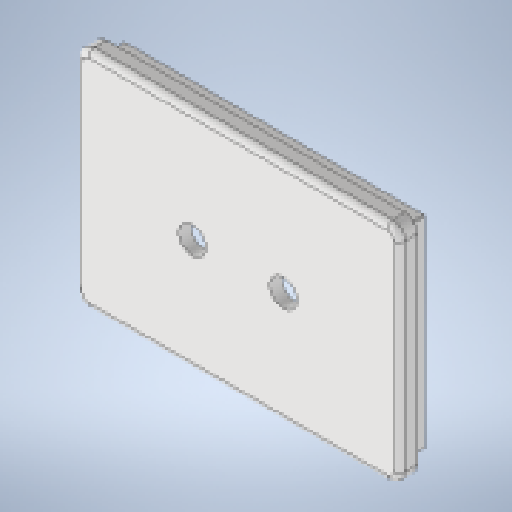
# Autodesk Inventor part: Frame_Bottom
Saved by Autodesk Inventor 2023 (Build 270158000, 158)
## iProperties
Created: 2023-10-08
Part Number: Frame_Bottom
Material: Generic
Document SubType Name: Modeling
Designer: a laptop
Density: 1 g/cm^3
Appearance: Default
Author: a laptop
Autodesk Inventor part; units mm, degrees
ref_plane "YZ Plane" through (0, 0, 0) normal (1, 0, 0) x (0, 1, 0)
ref_plane "XZ Plane" through (0, 0, 0) normal (0, 1, 0) x (-1, 0, 0)
ref_plane "XY Plane" through (0, 0, 0) normal (0, 0, 1) x (1, 0, 0)
sketch "Sketch1" plane through (0, 0, 0) normal (0, 0, 1) x (1, 0, 0)
  circle A0 centre (5, 5) radius 2.35
  line L0 (0, 0) -> (53.18, 0)
  line L1 (53.18, 0) -> (53.18, 36.924)
  line L2 (53.18, 36.924) -> (0, 36.924)
  line L3 (0, 36.924) -> (0, 0)
  circle A1 centre (5, 31.924) radius 2.35
  circle A2 centre (48.18, 5) radius 2.35
  circle A3 centre (48.18, 31.924) radius 2.35
  dimension "d0" = 5
  dimension "d1" = 5
  dimension "d4" = 26.924
  dimension "d7" = 43.18
  dimension "d10" = 5
  dimension "d11" = 5
  dimension "d12" = 4.7
  constraints: 8 end point, 4 centre point, 2 horizontal, 2 parallel, 1 perpendicular, 1 vertical, 6 other
  measures "d0" horizontal distance of L0.start A0.centre
  measures "d1" horizontal distance of L0.start A0.centre
  measures "d4" distance of A0.centre A1.centre
  measures "d7" distance of A0.centre A2.centre
  measures "d10" distance from line of L2 A3.centre
  measures "d11" distance from line of A3.centre L1
  measures "d12" diameter of A0
extrude "Extrusion1" add sketch "Sketch1" along normal blind 4
sketch "Sketch2" plane through (0, 0, 4) normal (0, 0, 1) x (1, 0, 0)
  line L0 (53.18, 0) -> (53.18, 36.924) projected
  line L1 (53.18, 36.924) -> (0, 36.924) projected
  line L2 (0, 36.924) -> (0, 0) projected
  line L3 (0, 0) -> (53.18, 0) projected
  circle A0 centre (5, 5) radius 2.35 projected
  circle A1 centre (5, 31.924) radius 2.35 projected
  circle A2 centre (48.18, 5) radius 2.35 projected
  circle A3 centre (48.18, 31.924) radius 2.35 projected
extrude "Extrusion2" add sketch "Sketch2" along normal blind 2 contours L3 L2 L1 L0 | A0 | A1 | A2 | A3
fillet "Fillet1" radius 2 4 edges at (53.18, 36.924, 3) (0, 36.924, 3) (53.18, 0, 3) (0, 0, 3)
sketch "Sketch3" plane through (0, 0, 0) normal (0, 0, -1) x (-1, 0, 0)
  line L0 (-41.59, 27.462) -> (-11.59, 27.462)
  line L1 (-11.59, 27.462) -> (-11.59, 9.462)
  line L2 (-11.59, 9.462) -> (-41.59, 9.462)
  line L3 (-41.59, 9.462) -> (-41.59, 27.462)
  line L4 (-51.18, 36.924) -> (-2, 36.924) projected
  line L5 (0, 34.924) -> (0, 2) projected
  line L6 (-26.59, 27.462) -> (-26.59, 36.924) construction
  line L7 (-11.59, 18.462) -> (0, 18.462) construction
  point P0 (0, 0)
  dimension "d18" = 30
  dimension "d19" = 18
  constraints: 12 end point, 4 midpoint, 2 horizontal, 2 parallel, 2 perpendicular
  measures "d18" distance of L0.start L0.end
  measures "d19" distance of L0.end L1.end
extrude "Extrusion3" cut sketch "Sketch3" against normal blind 4
fillet "Fillet2" radius 2 4 edges at (11.59, 27.462, 2) (41.59, 27.462, 2) (41.59, 9.462, 2) (11.59, 9.462, 2)
sketch "Sketch4" plane through (0, 0, 4) normal (0, 0, -1) x (-1, 0, 0)
  circle A0 centre (-19.09, 18.462) radius 2.2328
  circle A1 centre (-34.09, 18.462) radius 2.2328
  line L0 (-11.59, 25.462) -> (-11.59, 11.462) projected
  line L1 (-19.09, 18.462) -> (-34.09, 18.462) construction
  line L2 (-34.09, 18.462) -> (-26.59, 18.462) construction
  line L3 (-13.59, 9.462) -> (-39.59, 9.462) construction
  line L4 (-26.59, 9.462) -> (-26.59, 18.462) construction
  point P0 (0, 0)
  point P1 (-11.59, 18.462)
  dimension "d23" = 4.4656
  dimension "d24" = 15
  constraints: 6 end point, 3 midpoint, 2 centre point, 2 horizontal alignment, 1 equal radius, 1 horizontal, 1 perpendicular
  measures "d23" diameter of A0
  measures "d24" distance of L1.start L1.end
extrude "Extrusion4" cut sketch "Sketch4" against normal blind 3
fillet "Fillet3" radius 1 8 edges at (0.5858, 0.5858, 6) (26.59, 0, 6) (52.5942, 0.5858, 6) (53.18, 18.462, 6) (52.5942, 36.3382, 6) (26.59, 36.924, 6) (0.5858, 36.3382, 6) (0, 18.462, 6)
sketch "Sketch5" plane through (0, 0, 0) normal (0, 0, -1) x (-1, 0, 0)
  arc A0 (-51.18, 36.924) -> (-53.18, 34.924) centre (-51.18, 34.924) ccw projected
  line L0 (-53.18, 34.924) -> (-53.18, 2) projected
  arc A1 (-53.18, 2) -> (-51.18, 0) centre (-51.18, 2) ccw projected
  line L1 (-51.18, 0) -> (-2, 0) projected
  arc A2 (-2, 0) -> (0, 2) centre (-2, 2) ccw projected
  line L2 (0, 2) -> (0, 34.924) projected
  line L3 (-2, 36.924) -> (-51.18, 36.924) projected
  arc A3 (0, 34.924) -> (-2, 36.924) centre (-2, 34.924) ccw projected
  arc A4 (-1.6, 34.924) -> (-2, 35.324) centre (-2, 34.924) ccw projected
  line L4 (-2, 35.324) -> (-51.18, 35.324) projected
  arc A5 (-51.18, 35.324) -> (-51.58, 34.924) centre (-51.18, 34.924) ccw projected
  line L5 (-51.58, 34.924) -> (-51.58, 2) projected
  arc A6 (-51.58, 2) -> (-51.18, 1.6) centre (-51.18, 2) ccw projected
  line L6 (-51.18, 1.6) -> (-2, 1.6) projected
  arc A7 (-2, 1.6) -> (-1.6, 2) centre (-2, 2) ccw projected
  line L7 (-1.6, 2) -> (-1.6, 34.924) projected
  line L8 (0, 34.924) -> (0, 2) projected
  arc A8 (-2, 0) -> (0, 2) centre (-2, 2) ccw projected
  line L9 (-2, 0) -> (-51.18, 0) projected
  arc A9 (-53.18, 2) -> (-51.18, 0) centre (-51.18, 2) ccw projected
  line L10 (-53.18, 2) -> (-53.18, 34.924) projected
  arc A10 (-51.18, 36.924) -> (-53.18, 34.924) centre (-51.18, 34.924) ccw projected
  line L11 (-51.18, 36.924) -> (-2, 36.924) projected
  arc A11 (0, 34.924) -> (-2, 36.924) centre (-2, 34.924) ccw projected
  point P0 (0, 0)
extrude "Extrusion5" cut sketch "Sketch5" against normal blind 3
thicken "Thicken1" operation cut thickness 0.2 both sides no extend neighbours no toward (0, -1, 0) faces at (34.7867, 35.324, 1) (51.5105, 35.1493, 2) (51.58, 12.9747, 1) (51.3261, 1.6277, 2) (18.3933, 1.6, 1) (1.6277, 1.8539, 2) (1.6, 23.9493, 1) (1.7068, 35.1961, 2)
body "Solid1"
